Autodesk Fusion 360 part; units mm, degrees
note: some values were not read from the file. Set by a fixed rule: the direction of a hole.
(part 5 of 10)
  line L3822 (47.9298, 29.8196) -> (47.5996, 30.1498)
  line L3823 (47.9298, 31.1404) -> (48.5902, 31.1404)
  line L3824 (48.5902, 29.8196) -> (47.9298, 29.8196)
  line L3825 (48.9204, 30.8102) -> (48.9204, 30.1498)
  line L3826 (48.9204, 30.1498) -> (48.5902, 29.8196)
  line L3827 (48.5902, 31.1404) -> (48.9204, 30.8102)
  line L3828 (52.6796, 20.6502) -> (53.0098, 20.9804)
  line L3829 (53.6702, 19.6596) -> (53.0098, 19.6596)
  line L3830 (52.6796, 19.9898) -> (52.6796, 20.6502)
  line L3831 (54.0004, 20.6502) -> (54.0004, 19.9898)
  line L3832 (53.0098, 20.9804) -> (53.6702, 20.9804)
  line L3833 (53.0098, 19.6596) -> (52.6796, 19.9898)
  line L3834 (53.6702, 20.9804) -> (54.0004, 20.6502)
  line L3835 (54.0004, 19.9898) -> (53.6702, 19.6596)
  line L3836 (53.0098, 31.1404) -> (53.6702, 31.1404)
  line L3837 (54.0004, 30.1498) -> (53.6702, 29.8196)
  line L3838 (54.0004, 30.8102) -> (54.0004, 30.1498)
  line L3839 (53.6702, 31.1404) -> (54.0004, 30.8102)
  line L3840 (52.6796, 30.8102) -> (53.0098, 31.1404)
  line L3841 (53.0098, 29.8196) -> (52.6796, 30.1498)
  line L3842 (52.6796, 30.1498) -> (52.6796, 30.8102)
  line L3843 (53.6702, 29.8196) -> (53.0098, 29.8196)
  line L3844 (66.6496, 19.9898) -> (66.6496, 20.6502)
  line L3845 (67.6402, 20.9804) -> (67.9704, 20.6502)
  line L3846 (67.9704, 20.6502) -> (67.9704, 19.9898)
  line L3847 (67.9704, 19.9898) -> (67.6402, 19.6596)
  line L3848 (66.6496, 20.6502) -> (66.9798, 20.9804)
  line L3849 (66.9798, 19.6596) -> (66.6496, 19.9898)
  line L3850 (67.6402, 19.6596) -> (66.9798, 19.6596)
  line L3851 (66.9798, 20.9804) -> (67.6402, 20.9804)
  line L3852 (66.9798, 31.1404) -> (67.6402, 31.1404)
  line L3853 (67.9704, 30.8102) -> (67.9704, 30.1498)
  line L3854 (67.6402, 31.1404) -> (67.9704, 30.8102)
  line L3855 (66.9798, 29.8196) -> (66.6496, 30.1498)
  line L3856 (67.9704, 30.1498) -> (67.6402, 29.8196)
  line L3857 (66.6496, 30.1498) -> (66.6496, 30.8102)
  line L3858 (66.6496, 30.8102) -> (66.9798, 31.1404)
  line L3859 (67.6402, 29.8196) -> (66.9798, 29.8196)
  line L3860 (78.4098, 20.9804) -> (79.0702, 20.9804)
  line L3861 (79.4004, 19.9898) -> (79.0702, 19.6596)
  line L3862 (79.0702, 19.6596) -> (78.4098, 19.6596)
  line L3863 (79.0702, 20.9804) -> (79.4004, 20.6502)
  line L3864 (79.4004, 20.6502) -> (79.4004, 19.9898)
  line L3865 (78.4098, 19.6596) -> (78.0796, 19.9898)
  line L3866 (78.0796, 19.9898) -> (78.0796, 20.6502)
  line L3867 (78.0796, 20.6502) -> (78.4098, 20.9804)
  line L3868 (79.0702, 29.8196) -> (78.4098, 29.8196)
  line L3869 (79.0702, 31.1404) -> (79.4004, 30.8102)
  line L3870 (79.4004, 30.8102) -> (79.4004, 30.1498)
  line L3871 (78.4098, 29.8196) -> (78.0796, 30.1498)
  line L3872 (78.0796, 30.8102) -> (78.4098, 31.1404)
  line L3873 (78.4098, 31.1404) -> (79.0702, 31.1404)
  line L3874 (79.4004, 30.1498) -> (79.0702, 29.8196)
  line L3875 (78.0796, 30.1498) -> (78.0796, 30.8102)
  line L3876 (90.5002, 19.6596) -> (89.8398, 19.6596)
  line L3877 (90.8304, 19.9898) -> (90.5002, 19.6596)
  line L3878 (89.5096, 19.9898) -> (89.5096, 20.6502)
  line L3879 (89.8398, 20.9804) -> (90.5002, 20.9804)
  line L3880 (90.5002, 20.9804) -> (90.8304, 20.6502)
  line L3881 (89.8398, 19.6596) -> (89.5096, 19.9898)
  line L3882 (90.8304, 20.6502) -> (90.8304, 19.9898)
  line L3883 (89.5096, 20.6502) -> (89.8398, 20.9804)
  line L3884 (89.5096, 30.1498) -> (89.5096, 30.8102)
  line L3885 (89.5096, 30.8102) -> (89.8398, 31.1404)
  line L3886 (89.8398, 31.1404) -> (90.5002, 31.1404)
  line L3887 (90.8304, 30.8102) -> (90.8304, 30.1498)
  line L3888 (90.8304, 30.1498) -> (90.5002, 29.8196)
  line L3889 (90.5002, 29.8196) -> (89.8398, 29.8196)
  line L3890 (89.8398, 29.8196) -> (89.5096, 30.1498)
  line L3891 (90.5002, 31.1404) -> (90.8304, 30.8102)
  line L3892 (34.7234, 76.3657) -> (34.2565, 76.8326)
  line L3893 (35.6574, 76.8326) -> (35.1904, 76.3657)
  line L3894 (34.2565, 76.8326) -> (34.2565, 77.2996)
  line L3895 (35.1904, 77.7666) -> (35.6574, 77.2996)
  line L3896 (35.1904, 76.3657) -> (34.7234, 76.3657)
  line L3897 (34.2565, 77.2996) -> (34.7234, 77.7666)
  line L3898 (34.7234, 77.7666) -> (35.1904, 77.7666)
  line L3899 (35.6574, 77.2996) -> (35.6574, 76.8326)
  line L3900 (41.9076, 69.1815) -> (41.4407, 69.6484)
  line L3901 (41.4407, 69.6484) -> (41.4407, 70.1154)
  line L3902 (42.3746, 70.5824) -> (42.8416, 70.1154)
  line L3903 (42.8416, 70.1154) -> (42.8416, 69.6484)
  line L3904 (42.3746, 69.1815) -> (41.9076, 69.1815)
  line L3905 (41.4407, 70.1154) -> (41.9076, 70.5824)
  line L3906 (42.8416, 69.6484) -> (42.3746, 69.1815)
  line L3907 (41.9076, 70.5824) -> (42.3746, 70.5824)
  line L3908 (28.5496, 77.1652) -> (28.8798, 77.4954)
  line L3909 (28.8798, 76.1746) -> (28.5496, 76.5048)
  line L3910 (28.8798, 77.4954) -> (29.5402, 77.4954)
  line L3911 (28.5496, 76.5048) -> (28.5496, 77.1652)
  line L3912 (29.8704, 77.1652) -> (29.8704, 76.5048)
  line L3913 (29.5402, 76.1746) -> (28.8798, 76.1746)
  line L3914 (29.5402, 77.4954) -> (29.8704, 77.1652)
  line L3915 (29.8704, 76.5048) -> (29.5402, 76.1746)
  line L3916 (27.0002, 76.1746) -> (26.3398, 76.1746)
  line L3917 (26.3398, 76.1746) -> (26.0096, 76.5048)
  line L3918 (27.3304, 76.5048) -> (27.0002, 76.1746)
  line L3919 (26.0096, 77.1652) -> (26.3398, 77.4954)
  line L3920 (26.3398, 77.4954) -> (27.0002, 77.4954)
  line L3921 (27.0002, 77.4954) -> (27.3304, 77.1652)
  line L3922 (27.3304, 77.1652) -> (27.3304, 76.5048)
  line L3923 (26.0096, 76.5048) -> (26.0096, 77.1652)
  line L3924 (88.265, 70.485) -> (75.565, 57.785)
  line L3925 (98.425, 37.465) -> (98.425, 70.485)
  line L3926 (52.07, 57.785) -> (52.07, 37.465)
  line L3927 (75.565, 57.785) -> (52.07, 57.785)
  line L3928 (52.07, 37.465) -> (98.425, 37.465)
  line L3929 (98.425, 70.485) -> (88.265, 70.485)
  line L3930 (1.27, 71.12) -> (10.795, 71.12)
  line L3931 (1.27, 37.465) -> (1.27, 71.12)
  line L3932 (10.795, 71.12) -> (24.13, 57.785)
  line L3933 (48.895, 57.785) -> (48.895, 37.465)
  line L3934 (48.895, 37.465) -> (1.27, 37.465)
  line L3935 (24.13, 57.785) -> (48.895, 57.785)
  line L3936 (74.295, 70.485) -> (66.04, 78.74)
  line L3937 (26.035, 59.69) -> (74.295, 59.69)
  line L3938 (74.295, 59.69) -> (74.295, 70.485)
  line L3939 (66.04, 78.74) -> (34.29, 78.74)
  line L3940 (34.29, 78.74) -> (26.035, 70.485)
  line L3941 (26.035, 70.485) -> (26.035, 59.69)
  line L3942 (52.1716, 57.6834) -> (75.565, 57.6834)
  line L3943 (75.565, 57.6834) -> (75.6039, 57.6911)
  line L3944 (95.575, 66.9873) -> (95.3582, 66.5617)
  line L3945 (97.8163, 62.4021) -> (98.1561, 62.83)
  line L3946 (96.81, 67.6165) -> (96.3383, 67.5418)
  line L3947 (75.6039, 57.6911) -> (75.6368, 57.7132)
  line L3948 (96.3383, 67.5418) -> (95.9127, 67.325)
  line L3949 (95.2835, 66.09) -> (95.2835, 66.09)
  line L3950 (52.1716, 37.5666) -> (52.1716, 57.6834)
  line L3951 (95.2835, 63.55) -> (95.2835, 63.55)
  line L3952 (88.3071, 70.3834) -> (98.3234, 70.3834)
  line L3953 (98.1561, 66.81) -> (97.8163, 67.2379)
  line L3954 (98.3234, 63.3501) -> (98.3234, 37.5666)
  line L3955 (98.1561, 62.83) -> (98.3234, 63.3501)
  line L3956 (95.2835, 66.09) -> (95.2835, 63.55)
  line L3957 (75.6368, 57.7132) -> (88.3071, 70.3834)
  line L3958 (95.3582, 66.5617) -> (95.2835, 66.09)
  line L3959 (95.9127, 62.315) -> (96.3383, 62.0982)
  line L3960 (95.3582, 63.0783) -> (95.575, 62.6527)
  line L3961 (96.3383, 62.0982) -> (96.81, 62.0235)
  line L3962 (95.2835, 63.55) -> (95.3582, 63.0783)
  line L3963 (98.3234, 37.5666) -> (52.1716, 37.5666)
  line L3964 (97.8163, 67.2379) -> (97.3476, 67.5188)
  line L3965 (97.3476, 62.1212) -> (97.8163, 62.4021)
  line L3966 (98.3234, 70.3834) -> (98.3234, 66.2899)
  line L3967 (98.3234, 66.2899) -> (98.1561, 66.81)
  line L3968 (75.6368, 57.7132) -> (75.6368, 57.7132)
  line L3969 (97.3476, 67.5188) -> (96.81, 67.6165)
  line L3970 (95.575, 62.6527) -> (95.9127, 62.315)
  line L3971 (95.9127, 67.325) -> (95.575, 66.9873)
  line L3972 (96.81, 62.0235) -> (97.3476, 62.1212)
  line L3973 (95.813, 56.2555) -> (95.813, 56.2555)
  line L3974 (93.273, 56.2555) -> (93.273, 56.2555)
  line L3975 (92.038, 55.6263) -> (91.8212, 55.2007)
  line L3976 (95.813, 53.2025) -> (96.2847, 53.2772)
  line L3977 (92.3757, 55.964) -> (92.038, 55.6263)
  line L3978 (91.8212, 54.2573) -> (92.038, 53.8317)
  line L3979 (93.273, 53.2025) -> (93.273, 53.2025)
  line L3980 (95.813, 53.2025) -> (95.813, 53.2025)
  line L3981 (96.7103, 55.964) -> (96.2847, 56.1808)
  line L3982 (91.7465, 54.729) -> (91.8212, 54.2573)
  line L3983 (95.813, 56.2555) -> (93.273, 56.2555)
  line L3984 (91.8212, 55.2007) -> (91.7465, 54.729)
  line L3985 (96.7103, 53.494) -> (97.048, 53.8317)
  line L3986 (92.8013, 56.1808) -> (92.3757, 55.964)
  line L3987 (97.2648, 55.2007) -> (97.048, 55.6263)
  line L3988 (97.2648, 54.2573) -> (97.3395, 54.729)
  line L3989 (93.273, 53.2025) -> (95.813, 53.2025)
  line L3990 (92.8013, 53.2772) -> (93.273, 53.2025)
  line L3991 (96.2847, 56.1808) -> (95.813, 56.2555)
  line L3992 (92.3757, 53.494) -> (92.8013, 53.2772)
  line L3993 (97.3395, 54.729) -> (97.2648, 55.2007)
  line L3994 (96.2847, 53.2772) -> (96.7103, 53.494)
  line L3995 (97.048, 55.6263) -> (96.7103, 55.964)
  line L3996 (93.273, 56.2555) -> (92.8013, 56.1808)
  line L3997 (97.048, 53.8317) -> (97.2648, 54.2573)
  line L3998 (92.038, 53.8317) -> (92.3757, 53.494)
  line L3999 (71.5197, 53.2772) -> (71.9453, 53.494)
  line L4000 (71.048, 53.2025) -> (71.5197, 53.2772)
  line L4001 (71.048, 53.2025) -> (71.048, 53.2025)
  line L4002 (71.5197, 56.1808) -> (71.048, 56.2555)
  line L4003 (68.0363, 53.2772) -> (68.508, 53.2025)
  line L4004 (67.0562, 54.2573) -> (67.273, 53.8317)
  line L4005 (67.6107, 55.964) -> (67.273, 55.6263)
  line L4006 (68.508, 56.2555) -> (68.0363, 56.1808)
  line L4007 (72.283, 53.8317) -> (72.4998, 54.2573)
  line L4008 (72.4998, 55.2007) -> (72.283, 55.6263)
  line L4009 (72.4998, 54.2573) -> (72.5745, 54.729)
  line L4010 (71.048, 56.2555) -> (68.508, 56.2555)
  line L4011 (72.5745, 54.729) -> (72.4998, 55.2007)
  line L4012 (71.9453, 53.494) -> (72.283, 53.8317)
  line L4013 (67.273, 53.8317) -> (67.6107, 53.494)
  line L4014 (66.9815, 54.729) -> (67.0562, 54.2573)
  line L4015 (68.508, 53.2025) -> (68.508, 53.2025)
  line L4016 (72.283, 55.6263) -> (71.9453, 55.964)
  line L4017 (71.048, 56.2555) -> (71.048, 56.2555)
  line L4018 (67.273, 55.6263) -> (67.0562, 55.2007)
  line L4019 (67.0562, 55.2007) -> (66.9815, 54.729)
  line L4020 (68.0363, 56.1808) -> (67.6107, 55.964)
  line L4021 (67.6107, 53.494) -> (68.0363, 53.2772)
  line L4022 (68.508, 56.2555) -> (68.508, 56.2555)
  line L4023 (68.508, 53.2025) -> (71.048, 53.2025)
  line L4024 (71.9453, 55.964) -> (71.5197, 56.1808)
  line L4025 (79.7562, 54.2573) -> (79.973, 53.8317)
  line L4026 (84.6453, 55.964) -> (84.2197, 56.1808)
  line L4027 (85.1998, 54.2573) -> (85.2745, 54.729)
  line L4028 (83.748, 53.2025) -> (84.2197, 53.2772)
  line L4029 (84.983, 53.8317) -> (85.1998, 54.2573)
  line L4030 (81.208, 56.2555) -> (80.7363, 56.1808)
  line L4031 (80.7363, 53.2772) -> (81.208, 53.2025)
  line L4032 (80.3107, 53.494) -> (80.7363, 53.2772)
  line L4033 (84.983, 55.6263) -> (84.6453, 55.964)
  line L4034 (81.208, 56.2555) -> (81.208, 56.2555)
  line L4035 (81.208, 53.2025) -> (81.208, 53.2025)
  line L4036 (79.973, 53.8317) -> (80.3107, 53.494)
  line L4037 (79.7562, 55.2007) -> (79.6815, 54.729)
  line L4038 (81.208, 53.2025) -> (83.748, 53.2025)
  line L4039 (83.748, 53.2025) -> (83.748, 53.2025)
  line L4040 (79.6815, 54.729) -> (79.7562, 54.2573)
  line L4041 (84.2197, 56.1808) -> (83.748, 56.2555)
  line L4042 (85.1998, 55.2007) -> (84.983, 55.6263)
  line L4043 (83.748, 56.2555) -> (81.208, 56.2555)
  line L4044 (80.7363, 56.1808) -> (80.3107, 55.964)
  line L4045 (84.6453, 53.494) -> (84.983, 53.8317)
  line L4046 (80.3107, 55.964) -> (79.973, 55.6263)
  line L4047 (83.748, 56.2555) -> (83.748, 56.2555)
  line L4048 (79.973, 55.6263) -> (79.7562, 55.2007)
  line L4049 (84.2197, 53.2772) -> (84.6453, 53.494)
  line L4050 (85.2745, 54.729) -> (85.1998, 55.2007)
  line L4051 (58.348, 56.2555) -> (58.348, 56.2555)
  line L4052 (59.583, 55.6263) -> (59.2453, 55.964)
  line L4053 (55.3363, 53.2772) -> (55.808, 53.2025)
  line L4054 (54.3562, 54.2573) -> (54.573, 53.8317)
  line L4055 (55.808, 56.2555) -> (55.3363, 56.1808)
  line L4056 (58.348, 53.2025) -> (58.348, 53.2025)
  line L4057 (59.7998, 55.2007) -> (59.583, 55.6263)
  line L4058 (59.8745, 54.729) -> (59.7998, 55.2007)
  line L4059 (59.583, 53.8317) -> (59.7998, 54.2573)
  line L4060 (59.2453, 53.494) -> (59.583, 53.8317)
  line L4061 (58.8197, 53.2772) -> (59.2453, 53.494)
  line L4062 (58.348, 53.2025) -> (58.8197, 53.2772)
  line L4063 (55.808, 53.2025) -> (55.808, 53.2025)
  line L4064 (59.7998, 54.2573) -> (59.8745, 54.729)
  line L4065 (54.573, 55.6263) -> (54.3562, 55.2007)
  line L4066 (59.2453, 55.964) -> (58.8197, 56.1808)
  line L4067 (58.348, 56.2555) -> (55.808, 56.2555)
  line L4068 (55.808, 56.2555) -> (55.808, 56.2555)
  line L4069 (54.573, 53.8317) -> (54.9107, 53.494)
  line L4070 (55.808, 53.2025) -> (58.348, 53.2025)
  line L4071 (58.8197, 56.1808) -> (58.348, 56.2555)
  line L4072 (54.3562, 55.2007) -> (54.2815, 54.729)
  line L4073 (54.9107, 53.494) -> (55.3363, 53.2772)
  line L4074 (54.2815, 54.729) -> (54.3562, 54.2573)
  line L4075 (54.9107, 55.964) -> (54.573, 55.6263)
  line L4076 (55.3363, 56.1808) -> (54.9107, 55.964)
  line L4077 (1.3716, 71.0184) -> (10.7529, 71.0184)
  line L4078 (48.7934, 57.6834) -> (48.7934, 37.5666)
  line L4079 (24.0582, 57.7132) -> (24.0582, 57.7132)
  line L4080 (24.13, 57.6834) -> (48.7934, 57.6834)
  line L4081 (24.0911, 57.6911) -> (24.13, 57.6834)
  line L4082 (1.3716, 37.5666) -> (1.3716, 71.0184)
  line L4083 (24.0582, 57.7132) -> (24.0911, 57.6911)
  line L4084 (48.7934, 37.5666) -> (1.3716, 37.5666)
  line L4085 (10.7529, 71.0184) -> (24.0582, 57.7132)
  line L4086 (2.9212, 54.2573) -> (3.138, 53.8317)
  line L4087 (3.9013, 53.2772) -> (4.373, 53.2025)
  line L4088 (6.913, 53.2025) -> (7.3847, 53.2772)
  line L4089 (3.138, 53.8317) -> (3.4757, 53.494)
  line L4090 (2.8465, 54.729) -> (2.9212, 54.2573)
  line L4091 (4.373, 53.2025) -> (4.373, 53.2025)
  line L4092 (3.9013, 56.1808) -> (3.4757, 55.964)
  line L4093 (3.138, 55.6263) -> (2.9212, 55.2007)
  line L4094 (7.3847, 56.1808) -> (6.913, 56.2555)
  line L4095 (3.4757, 53.494) -> (3.9013, 53.2772)
  line L4096 (2.9212, 55.2007) -> (2.8465, 54.729)
  line L4097 (6.913, 53.2025) -> (6.913, 53.2025)
  line L4098 (7.8103, 53.494) -> (8.148, 53.8317)
  line L4099 (6.913, 56.2555) -> (4.373, 56.2555)
  line L4100 (8.3648, 55.2007) -> (8.148, 55.6263)
  line L4101 (8.148, 55.6263) -> (7.8103, 55.964)
  line L4102 (7.8103, 55.964) -> (7.3847, 56.1808)
  line L4103 (8.148, 53.8317) -> (8.3648, 54.2573)
  line L4104 (6.913, 56.2555) -> (6.913, 56.2555)
  line L4105 (3.4757, 55.964) -> (3.138, 55.6263)
  line L4106 (8.3648, 54.2573) -> (8.4395, 54.729)
  line L4107 (4.373, 56.2555) -> (3.9013, 56.1808)
  line L4108 (4.373, 56.2555) -> (4.373, 56.2555)
  line L4109 (7.3847, 53.2772) -> (7.8103, 53.494)
  line L4110 (4.373, 53.2025) -> (6.913, 53.2025)
  line L4111 (8.4395, 54.729) -> (8.3648, 55.2007)
  line L4112 (20.848, 55.6263) -> (20.5103, 55.964)
  line L4113 (21.1395, 54.729) -> (21.0648, 55.2007)
  line L4114 (20.5103, 55.964) -> (20.0847, 56.1808)
  line L4115 (20.0847, 56.1808) -> (19.613, 56.2555)
  line L4116 (19.613, 56.2555) -> (19.613, 56.2555)
  line L4117 (20.848, 53.8317) -> (21.0648, 54.2573)
  line L4118 (21.0648, 54.2573) -> (21.1395, 54.729)
  line L4119 (15.6212, 54.2573) -> (15.838, 53.8317)
  line L4120 (19.613, 56.2555) -> (17.073, 56.2555)
  line L4121 (17.073, 56.2555) -> (17.073, 56.2555)
  line L4122 (15.5465, 54.729) -> (15.6212, 54.2573)
  line L4123 (15.838, 55.6263) -> (15.6212, 55.2007)
  line L4124 (21.0648, 55.2007) -> (20.848, 55.6263)
  line L4125 (16.1757, 55.964) -> (15.838, 55.6263)
  line L4126 (16.6013, 53.2772) -> (17.073, 53.2025)
  line L4127 (17.073, 56.2555) -> (16.6013, 56.1808)
  line L4128 (16.1757, 53.494) -> (16.6013, 53.2772)
  line L4129 (15.6212, 55.2007) -> (15.5465, 54.729)
  line L4130 (17.073, 53.2025) -> (17.073, 53.2025)
  line L4131 (19.613, 53.2025) -> (20.0847, 53.2772)
  line L4132 (19.613, 53.2025) -> (19.613, 53.2025)
  line L4133 (15.838, 53.8317) -> (16.1757, 53.494)
  line L4134 (16.6013, 56.1808) -> (16.1757, 55.964)
  line L4135 (17.073, 53.2025) -> (19.613, 53.2025)
  line L4136 (20.5103, 53.494) -> (20.848, 53.8317)
  line L4137 (20.0847, 53.2772) -> (20.5103, 53.494)
  line L4138 (32.7847, 53.2772) -> (33.2103, 53.494)
  line L4139 (33.2103, 53.494) -> (33.548, 53.8317)
  line L4140 (33.548, 55.6263) -> (33.2103, 55.964)
  line L4141 (29.773, 53.2025) -> (29.773, 53.2025)
  line L4142 (32.313, 53.2025) -> (32.313, 53.2025)
  line L4143 (29.773, 56.2555) -> (29.3013, 56.1808)
  line L4144 (32.7847, 56.1808) -> (32.313, 56.2555)
  line L4145 (28.538, 53.8317) -> (28.8757, 53.494)
  line L4146 (32.313, 56.2555) -> (29.773, 56.2555)
  line L4147 (28.8757, 55.964) -> (28.538, 55.6263)
  line L4148 (28.8757, 53.494) -> (29.3013, 53.2772)
  line L4149 (33.548, 53.8317) -> (33.7648, 54.2573)
  line L4150 (28.3212, 55.2007) -> (28.2465, 54.729)
  line L4151 (32.313, 56.2555) -> (32.313, 56.2555)
  line L4152 (33.7648, 55.2007) -> (33.548, 55.6263)
  line L4153 (33.2103, 55.964) -> (32.7847, 56.1808)
  line L4154 (29.3013, 56.1808) -> (28.8757, 55.964)
  line L4155 (28.3212, 54.2573) -> (28.538, 53.8317)
  line L4156 (32.313, 53.2025) -> (32.7847, 53.2772)
  line L4157 (29.773, 56.2555) -> (29.773, 56.2555)
  line L4158 (33.7648, 54.2573) -> (33.8395, 54.729)
  line L4159 (33.8395, 54.729) -> (33.7648, 55.2007)
  line L4160 (28.538, 55.6263) -> (28.3212, 55.2007)
  line L4161 (28.2465, 54.729) -> (28.3212, 54.2573)
  line L4162 (29.3013, 53.2772) -> (29.773, 53.2025)
  line L4163 (29.773, 53.2025) -> (32.313, 53.2025)
  line L4164 (4.9718, 62.9783) -> (5.0465, 63.45)
  line L4165 (4.755, 62.5527) -> (4.9718, 62.9783)
  line L4166 (4.4173, 62.215) -> (4.755, 62.5527)
  line L4167 (3.9917, 61.9982) -> (4.4173, 62.215)
  line L4168 (3.0483, 61.9982) -> (3.52, 61.9235)
  line L4169 (3.52, 67.5165) -> (3.0483, 67.4418)
  line L4170 (5.0465, 63.45) -> (5.0465, 63.45)
  line L4171 (3.9917, 67.4418) -> (3.52, 67.5165)
  line L4172 (5.0465, 63.45) -> (5.0465, 65.99)
  line L4173 (3.52, 61.9235) -> (3.9917, 61.9982)
  line L4174 (1.9935, 63.45) -> (2.0682, 62.9783)
  line L4175 (5.0465, 65.99) -> (5.0465, 65.99)
  line L4176 (2.6227, 62.215) -> (3.0483, 61.9982)
  line L4177 (3.0483, 67.4418) -> (2.6227, 67.225)
  line L4178 (2.285, 62.5527) -> (2.6227, 62.215)
  line L4179 (4.4173, 67.225) -> (3.9917, 67.4418)
  line L4180 (1.9935, 63.45) -> (1.9935, 63.45)
  line L4181 (5.0465, 65.99) -> (4.9718, 66.4617)
  line L4182 (2.0682, 62.9783) -> (2.285, 62.5527)
  line L4183 (4.9718, 66.4617) -> (4.755, 66.8873)
  line L4184 (2.0682, 66.4617) -> (1.9935, 65.99)
  line L4185 (4.755, 66.8873) -> (4.4173, 67.225)
  line L4186 (2.285, 66.8873) -> (2.0682, 66.4617)
  line L4187 (1.9935, 65.99) -> (1.9935, 63.45)
  line L4188 (2.6227, 67.225) -> (2.285, 66.8873)
  line L4189 (1.9935, 65.99) -> (1.9935, 65.99)
  line L4190 (45.013, 56.2555) -> (45.013, 56.2555)
  line L4191 (45.013, 53.2025) -> (45.013, 53.2025)
  line L4192 (41.0212, 55.2007) -> (40.9465, 54.729)
  line L4193 (41.238, 53.8317) -> (41.5757, 53.494)
  line L4194 (46.5395, 54.729) -> (46.4648, 55.2007)
  line L4195 (42.473, 56.2555) -> (42.473, 56.2555)
  line L4196 (41.0212, 54.2573) -> (41.238, 53.8317)
  line L4197 (40.9465, 54.729) -> (41.0212, 54.2573)
  line L4198 (42.0013, 56.1808) -> (41.5757, 55.964)
  line L4199 (46.4648, 54.2573) -> (46.5395, 54.729)
  line L4200 (46.4648, 55.2007) -> (46.248, 55.6263)
  line L4201 (41.5757, 53.494) -> (42.0013, 53.2772)
  line L4202 (41.238, 55.6263) -> (41.0212, 55.2007)
  line L4203 (41.5757, 55.964) -> (41.238, 55.6263)
  line L4204 (46.248, 55.6263) -> (45.9103, 55.964)
  line L4205 (42.473, 53.2025) -> (45.013, 53.2025)
  line L4206 (45.4847, 53.2772) -> (45.9103, 53.494)
  line L4207 (42.473, 53.2025) -> (42.473, 53.2025)
  line L4208 (46.248, 53.8317) -> (46.4648, 54.2573)
  line L4209 (45.9103, 53.494) -> (46.248, 53.8317)
  line L4210 (42.0013, 53.2772) -> (42.473, 53.2025)
  line L4211 (42.473, 56.2555) -> (42.0013, 56.1808)
  line L4212 (45.013, 53.2025) -> (45.4847, 53.2772)
  line L4213 (45.9103, 55.964) -> (45.4847, 56.1808)
  line L4214 (45.013, 56.2555) -> (42.473, 56.2555)
  line L4215 (45.4847, 56.1808) -> (45.013, 56.2555)
  line L4216 (34.5864, 78.0975) -> (34.4702, 78.0198)
  line L4217 (34.0032, 77.5528) -> (34.0032, 77.5528)
  line L4218 (34.5864, 76.0348) -> (34.7234, 76.0075)
  line L4219 (26.1366, 59.7916) -> (26.1366, 70.4429)
  line L4220 (35.3275, 78.0975) -> (35.1904, 78.1247)
  line L4221 (34.4702, 78.0198) -> (34.4702, 78.0198)
  line L4222 (65.9979, 78.6384) -> (74.1934, 70.4429)
  line L4223 (35.9882, 76.6956) -> (36.0155, 76.8326)
  line L4224 (34.1819, 76.4007) -> (34.4702, 76.1124)
  line L4225 (36.0155, 77.2996) -> (35.9882, 77.4367)
  line L4226 (35.1904, 76.0075) -> (35.3275, 76.0348)
  line L4227 (35.9106, 77.5528) -> (35.4436, 78.0198)
  line L4228 (35.1904, 78.1247) -> (34.7234, 78.1247)
  line L4229 (26.1366, 70.4429) -> (32.0943, 76.4007)
  line L4230 (35.9106, 77.5528) -> (35.9106, 77.5528)
  line L4231 (35.4436, 78.0198) -> (35.3275, 78.0975)
  line L4232 (35.1904, 76.0075) -> (35.1904, 76.0075)
  line L4233 (34.4702, 76.1124) -> (34.4702, 76.1124)
  line L4234 (33.8983, 77.2996) -> (33.8983, 77.2996)
  line L4235 (34.7234, 76.0075) -> (34.7234, 76.0075)
  line L4236 (34.7234, 76.0075) -> (35.1904, 76.0075)
  line L4237 (36.0155, 77.2996) -> (36.0155, 77.2996)
  line L4238 (35.3275, 76.0348) -> (35.4436, 76.1124)
  line L4239 (74.1934, 59.7916) -> (26.1366, 59.7916)
  line L4240 (32.0943, 76.4007) -> (34.1819, 76.4007)
  line L4241 (74.1934, 70.4429) -> (74.1934, 59.7916)
  line L4242 (36.0155, 76.8326) -> (36.0155, 76.8326)
  line L4243 (34.4702, 76.1124) -> (34.5864, 76.0348)
  line L4244 (35.9106, 76.5794) -> (35.9106, 76.5794)
  line L4245 (35.4436, 78.0198) -> (35.4436, 78.0198)
  line L4246 (35.9882, 77.4367) -> (35.9106, 77.5528)
  line L4247 (33.9256, 77.4367) -> (33.8983, 77.2996)
  line L4248 (35.4436, 76.1124) -> (35.9106, 76.5794)
  line L4249 (34.4702, 78.0198) -> (34.0032, 77.5528)
  line L4250 (35.9106, 76.5794) -> (35.9882, 76.6956)
  line L4251 (33.8983, 77.2693) -> (32.963, 77.2693)
  line L4252 (36.0155, 76.8326) -> (36.0155, 77.2996)
  line L4253 (33.8983, 77.2996) -> (33.8983, 77.2693)
  line L4254 (32.963, 77.2693) -> (34.3321, 78.6384)
  line L4255 (34.0032, 77.5528) -> (33.9256, 77.4367)
  line L4256 (34.7234, 78.1247) -> (34.7234, 78.1247)
  line L4257 (35.1904, 78.1247) -> (35.1904, 78.1247)
  line L4258 (34.7234, 78.1247) -> (34.5864, 78.0975)
  line L4259 (34.3321, 78.6384) -> (65.9979, 78.6384)
  line L4260 (38.5465, 65.965) -> (38.4718, 66.4367)
  line L4261 (35.5682, 66.4367) -> (35.4935, 65.965)
  line L4262 (37.4917, 61.9732) -> (37.9173, 62.19)
  line L4263 (38.5465, 65.965) -> (38.5465, 65.965)
  line L4264 (36.1227, 67.2) -> (35.785, 66.8623)
  line L4265 (35.4935, 65.965) -> (35.4935, 63.425)
  line L4266 (38.255, 62.5277) -> (38.4718, 62.9533)
  line L4267 (37.02, 67.4915) -> (36.5483, 67.4168)
  line L4268 (36.5483, 61.9732) -> (37.02, 61.8985)
  line L4269 (35.4935, 63.425) -> (35.4935, 63.425)
  line L4270 (35.785, 66.8623) -> (35.5682, 66.4367)
  line L4271 (36.5483, 67.4168) -> (36.1227, 67.2)
  line L4272 (35.785, 62.5277) -> (36.1227, 62.19)
  line L4273 (35.4935, 65.965) -> (35.4935, 65.965)
  line L4274 (38.5465, 63.425) -> (38.5465, 63.425)
  line L4275 (35.4935, 63.425) -> (35.5682, 62.9533)
  line L4276 (38.5465, 63.425) -> (38.5465, 65.965)
  line L4277 (38.255, 66.8623) -> (37.9173, 67.2)
  line L4278 (37.4917, 67.4168) -> (37.02, 67.4915)
  line L4279 (36.1227, 62.19) -> (36.5483, 61.9732)
  line L4280 (38.4718, 62.9533) -> (38.5465, 63.425)
  line L4281 (37.9173, 62.19) -> (38.255, 62.5277)
  line L4282 (37.9173, 67.2) -> (37.4917, 67.4168)
  line L4283 (35.5682, 62.9533) -> (35.785, 62.5277)
  line L4284 (37.02, 61.8985) -> (37.4917, 61.9732)
  line L4285 (38.4718, 66.4367) -> (38.255, 66.8623)
  line L4286 (61.8582, 63.1033) -> (62.075, 62.6777)
  line L4287 (64.7618, 63.1033) -> (64.8365, 63.575)
  line L4288 (61.7835, 63.575) -> (61.8582, 63.1033)
  line L4289 (62.075, 62.6777) -> (62.4127, 62.34)
  line L4290 (63.31, 67.6415) -> (62.8383, 67.5668)
  line L4291 (63.7817, 67.5668) -> (63.31, 67.6415)
  line L4292 (61.7835, 66.115) -> (61.7835, 63.575)
  line L4293 (63.31, 62.0485) -> (63.7817, 62.1232)
  line L4294 (63.7817, 62.1232) -> (64.2073, 62.34)
  line L4295 (64.7618, 66.5867) -> (64.545, 67.0123)
  line L4296 (61.7835, 63.575) -> (61.7835, 63.575)
  line L4297 (64.2073, 67.35) -> (63.7817, 67.5668)
  line L4298 (62.4127, 67.35) -> (62.075, 67.0123)
  line L4299 (62.075, 67.0123) -> (61.8582, 66.5867)
  line L4300 (61.7835, 66.115) -> (61.7835, 66.115)
  line L4301 (64.545, 62.6777) -> (64.7618, 63.1033)
  line L4302 (64.545, 67.0123) -> (64.2073, 67.35)
  line L4303 (61.8582, 66.5867) -> (61.7835, 66.115)
  line L4304 (62.4127, 62.34) -> (62.8383, 62.1232)
  line L4305 (64.8365, 63.575) -> (64.8365, 66.115)
  line L4306 (64.8365, 66.115) -> (64.8365, 66.115)
  line L4307 (62.8383, 62.1232) -> (63.31, 62.0485)
  line L4308 (62.8383, 67.5668) -> (62.4127, 67.35)
  line L4309 (64.8365, 63.575) -> (64.8365, 63.575)
  line L4310 (64.2073, 62.34) -> (64.545, 62.6777)
  line L4311 (64.8365, 66.115) -> (64.7618, 66.5867)
  line L4312 (52.0008, 76.8601) -> (51.9319, 76.425)
  line L4313 (54.1677, 73.1858) -> (54.4792, 73.4973)
  line L4314 (54.4792, 77.2527) -> (54.1677, 77.5642)
  line L4315 (52.5123, 73.1858) -> (52.9049, 72.9858)
  line L4316 (52.9049, 72.9858) -> (53.34, 72.9169)
  line L4317 (54.7481, 76.425) -> (54.7481, 76.425)
  line L4318 (52.5123, 77.5642) -> (52.2008, 77.2527)
  line L4319 (54.7481, 74.325) -> (54.7481, 76.425)
  line L4320 (54.1677, 77.5642) -> (53.7751, 77.7642)
  line L4321 (51.9319, 76.425) -> (51.9319, 76.425)
  line L4322 (54.7481, 76.425) -> (54.6792, 76.8601)
  line L4323 (54.4792, 73.4973) -> (54.6792, 73.8899)
  line L4324 (51.9319, 74.325) -> (51.9319, 74.325)
  line L4325 (53.34, 72.9169) -> (53.7751, 72.9858)
  line L4326 (52.2008, 77.2527) -> (52.0008, 76.8601)
  line L4327 (51.9319, 76.425) -> (51.9319, 74.325)
  line L4328 (53.7751, 77.7642) -> (53.34, 77.8331)
  line L4329 (51.9319, 74.325) -> (52.0008, 73.8899)
  line L4330 (54.6792, 73.8899) -> (54.7481, 74.325)
  line L4331 (53.7751, 72.9858) -> (54.1677, 73.1858)
  line L4332 (52.2008, 73.4973) -> (52.5123, 73.1858)
  line L4333 (53.34, 77.8331) -> (52.9049, 77.7642)
  line L4334 (54.6792, 76.8601) -> (54.4792, 77.2527)
  line L4335 (52.0008, 73.8899) -> (52.2008, 73.4973)
  line L4336 (54.7481, 74.325) -> (54.7481, 74.325)
  line L4337 (52.9049, 77.7642) -> (52.5123, 77.5642)
  line L4338 (49.4671, 76.925) -> (49.1839, 77.3489)
  line L4339 (48.76, 77.6321) -> (48.26, 77.7315)
  line L4340 (47.3361, 77.3489) -> (47.0529, 76.925)
  line L4341 (46.9535, 76.425) -> (46.9535, 74.325)
  line L4342 (48.26, 73.0185) -> (48.76, 73.1179)
  line L4343 (49.5665, 74.325) -> (49.5665, 74.325)
  line L4344 (49.1839, 73.4011) -> (49.4671, 73.825)
  line L4345 (49.4671, 73.825) -> (49.5665, 74.325)
  line L4346 (48.26, 77.7315) -> (47.76, 77.6321)
  line L4347 (47.3361, 73.4011) -> (47.76, 73.1179)
  line L4348 (46.9535, 74.325) -> (46.9535, 74.325)
  line L4349 (46.9535, 76.425) -> (46.9535, 76.425)
  line L4350 (46.9535, 74.325) -> (47.0529, 73.825)
  line L4351 (47.0529, 73.825) -> (47.3361, 73.4011)
  line L4352 (47.76, 77.6321) -> (47.3361, 77.3489)
  line L4353 (47.0529, 76.925) -> (46.9535, 76.425)
  line L4354 (49.1839, 77.3489) -> (48.76, 77.6321)
  line L4355 (49.5665, 76.425) -> (49.5665, 76.425)
  line L4356 (47.76, 73.1179) -> (48.26, 73.0185)
  line L4357 (49.5665, 74.325) -> (49.5665, 76.425)
  line L4358 (48.76, 73.1179) -> (49.1839, 73.4011)
  line L4359 (49.5665, 76.425) -> (49.4671, 76.925)
  line L4360 (41.9076, 70.8389) -> (41.9076, 70.8389)
  line L4361 (41.1841, 70.1154) -> (41.1841, 69.6484)
  line L4362 (41.2593, 70.2968) -> (41.2593, 70.2968)
  line L4363 (43.0981, 69.6484) -> (43.0981, 69.6484)
  line L4364 (43.023, 70.2968) -> (43.023, 70.2968)
  line L4365 (42.556, 69) -> (43.023, 69.467)
  line L4366 (41.7262, 69) -> (41.8095, 68.9444)
  line L4367 (41.8095, 68.9444) -> (41.9076, 68.9249)
  line L4368 (41.8095, 70.8194) -> (41.7262, 70.7638)
  line L4369 (41.7262, 70.7638) -> (41.2593, 70.2968)
  line L4370 (43.0786, 69.5502) -> (43.0981, 69.6484)
  line L4371 (42.4728, 70.8194) -> (42.3746, 70.8389)
  line L4372 (43.0981, 70.1154) -> (43.0981, 70.1154)
  line L4373 (42.556, 70.7638) -> (42.556, 70.7638)
  line L4374 (41.9076, 68.9249) -> (41.9076, 68.9249)
  line L4375 (41.2593, 69.467) -> (41.7262, 69)
  line L4376 (41.2036, 70.2136) -> (41.1841, 70.1154)
  line L4377 (41.7262, 69) -> (41.7262, 69)
  line L4378 (42.3746, 68.9249) -> (42.4728, 68.9444)
  line L4379 (43.023, 69.467) -> (43.023, 69.467)
  line L4380 (43.0981, 70.1154) -> (43.0786, 70.2136)
  line L4381 (42.556, 69) -> (42.556, 69)
  line L4382 (41.2036, 69.5502) -> (41.2593, 69.467)
  line L4383 (43.023, 70.2968) -> (42.556, 70.7638)
  line L4384 (41.1841, 70.1154) -> (41.1841, 70.1154)
  line L4385 (43.0786, 70.2136) -> (43.023, 70.2968)
  line L4386 (41.1841, 69.6484) -> (41.1841, 69.6484)
  line L4387 (42.4728, 68.9444) -> (42.556, 69)
  line L4388 (41.9076, 70.8389) -> (41.8095, 70.8194)
  line L4389 (42.3746, 70.8389) -> (42.3746, 70.8389)
  line L4390 (41.9076, 68.9249) -> (42.3746, 68.9249)
  line L4391 (41.1841, 69.6484) -> (41.2036, 69.5502)
  line L4392 (42.3746, 70.8389) -> (41.9076, 70.8389)
  line L4393 (43.0981, 69.6484) -> (43.0981, 70.1154)
  line L4394 (41.7262, 70.7638) -> (41.7262, 70.7638)
  line L4395 (42.3746, 68.9249) -> (42.3746, 68.9249)
  line L4396 (42.556, 70.7638) -> (42.4728, 70.8194)
  line L4397 (41.2593, 69.467) -> (41.2593, 69.467)
  line L4398 (41.2593, 70.2968) -> (41.2036, 70.2136)
  line L4399 (43.023, 69.467) -> (43.0786, 69.5502)
  line L4400 (57.078, 54.729) -> (59.7755, 54.729)
  line L4401 (57.078, 54.729) -> (54.3805, 54.729)
  line L4402 (57.078, 54.729) -> (57.078, 53.3015)
  line L4403 (57.078, 54.729) -> (57.078, 56.1565)
  line L4404 (69.778, 54.729) -> (72.4755, 54.729)
  line L4405 (69.778, 54.729) -> (67.0805, 54.729)
  line L4406 (69.778, 54.729) -> (69.778, 53.3015)
  line L4407 (69.778, 54.729) -> (69.778, 56.1565)
  line L4408 (82.478, 54.729) -> (85.1755, 54.729)
  line L4409 (82.478, 54.729) -> (79.7805, 54.729)
  line L4410 (82.478, 54.729) -> (82.478, 53.3015)
  line L4411 (82.478, 54.729) -> (82.478, 56.1565)
  line L4412 (94.543, 54.729) -> (97.2405, 54.729)
  line L4413 (94.543, 54.729) -> (91.8455, 54.729)
  line L4414 (94.543, 54.729) -> (94.543, 53.3015)
  line L4415 (94.543, 54.729) -> (94.543, 56.1565)
  line L4416 (96.81, 64.82) -> (96.81, 67.5175)
  line L4417 (96.81, 64.82) -> (96.81, 62.1225)
  line L4418 (96.81, 64.82) -> (95.3825, 64.82)
  line L4419 (3.52, 64.72) -> (3.52, 62.0225)
  line L4420 (3.52, 64.72) -> (3.52, 67.4175)
  line L4421 (3.52, 64.72) -> (2.0925, 64.72)
  line L4422 (3.52, 64.72) -> (4.9475, 64.72)
  line L4423 (5.643, 54.729) -> (8.3405, 54.729)
  line L4424 (5.643, 54.729) -> (2.9455, 54.729)
  line L4425 (5.643, 54.729) -> (5.643, 53.3015)
  line L4426 (5.643, 54.729) -> (5.643, 56.1565)
  line L4427 (18.343, 54.729) -> (21.0405, 54.729)
  line L4428 (18.343, 54.729) -> (15.6455, 54.729)
  line L4429 (18.343, 54.729) -> (18.343, 53.3015)
  line L4430 (18.343, 54.729) -> (18.343, 56.1565)
  line L4431 (31.043, 54.729) -> (33.7405, 54.729)
  line L4432 (31.043, 54.729) -> (28.3455, 54.729)
  line L4433 (31.043, 54.729) -> (31.043, 53.3015)
  line L4434 (31.043, 54.729) -> (31.043, 56.1565)
  line L4435 (43.743, 54.729) -> (46.4405, 54.729)
  line L4436 (43.743, 54.729) -> (41.0455, 54.729)
  line L4437 (43.743, 54.729) -> (43.743, 53.3015)
  line L4438 (43.743, 54.729) -> (43.743, 56.1565)
  line L4439 (37.02, 64.695) -> (37.02, 61.9975)
  line L4440 (37.02, 64.695) -> (37.02, 67.3925)
  line L4441 (37.02, 64.695) -> (35.5925, 64.695)
  line L4442 (37.02, 64.695) -> (38.4475, 64.695)
  line L4443 (42.1411, 69.8819) -> (41.5628, 70.4602)
  line L4444 (42.1411, 69.8819) -> (42.7194, 69.3036)
  line L4445 (42.1411, 69.8819) -> (42.7194, 70.4602)
  line L4446 (42.1411, 69.8819) -> (41.5628, 69.3036)
  line L4447 (48.26, 75.375) -> (48.26, 77.6325)
  line L4448 (48.26, 75.375) -> (48.26, 73.1175)
  line L4449 (48.26, 75.375) -> (49.4675, 75.375)
  line L4450 (48.26, 75.375) -> (47.0525, 75.375)
  line L4451 (63.31, 64.845) -> (63.31, 67.5425)
  line L4452 (63.31, 64.845) -> (63.31, 62.1475)
  line L4453 (63.31, 64.845) -> (64.7375, 64.845)
  line L4454 (63.31, 64.845) -> (61.8825, 64.845)
  line L4455 (69.778, 54.729) -> (57.078, 54.729)
  line L4456 (82.478, 54.729) -> (69.778, 54.729)
  line L4457 (96.81, 64.82) -> (94.543, 62.553)
  line L4458 (94.543, 62.553) -> (94.543, 54.729)
  line L4459 (94.543, 54.729) -> (57.078, 54.729)
  line L4460 (91.44, 76.2) -> (91.44, 69.215)
  line L4461 (95.835, 64.82) -> (96.81, 64.82)
  line L4462 (91.44, 69.215) -> (95.835, 64.82)
  line L4463 (3.52, 64.72) -> (4.79, 64.72)
  line L4464 (5.643, 63.867) -> (4.79, 64.72)
  line L4465 (5.643, 63.867) -> (5.643, 54.729)
  line L4466 (43.743, 54.729) -> (31.043, 54.729)
  line L4467 (31.043, 54.729) -> (31.5468, 54.729)
  line L4468 (31.5468, 54.729) -> (18.343, 54.729)
  line L4469 (18.343, 54.729) -> (18.9738, 54.729)
  line L4470 (18.9738, 54.729) -> (5.643, 54.729)
  line L4471 (3.52, 64.72) -> (8.89, 70.09)
  line L4472 (8.89, 70.09) -> (8.89, 76.835)
  line L4473 (18.8802, 54.729) -> (18.343, 54.729)
  line L4474 (18.8802, 54.729) -> (18.9738, 54.6354)
  line L4475 (18.9738, 54.6354) -> (18.9738, 54.729)
  line L4476 (31.5468, 54.3696) -> (31.5468, 54.6354)
  line L4477 (31.5468, 54.6354) -> (31.5468, 54.729)
  line L4478 (31.5468, 54.3696) -> (31.043, 54.729)
  line L4479 (48.26, 75.375) -> (48.26, 66.04)
  line L4480 (48.26, 66.04) -> (46.915, 64.695)
  line L4481 (46.915, 64.695) -> (37.02, 64.695)
  line L4482 (63.31, 64.845) -> (49.455, 64.845)
  line L4483 (49.455, 64.845) -> (48.26, 66.04)
  line L4484 (63.31, 64.845) -> (36.535, 64.845)
  line L4485 (37.17, 64.845) -> (37.02, 64.695)
  line L4486 (40.27, 64.845) -> (37.17, 64.845)
  line L4487 (37.17, 64.845) -> (36.535, 64.845)
  line L4488 (48.26, 75.375) -> (48.26, 72.835)
  line L4489 (56.25, 64.845) -> (63.31, 64.845)
  line L4490 (37.02, 64.695) -> (37.02, 64.7608)
  line L4491 (37.02, 64.7608) -> (42.1411, 69.8819)
  line L4492 (78.74, 76.2) -> (81.28, 76.2)
  line L4493 (21.59, 76.835) -> (19.05, 76.835)
  line L4494 (4.635, 15.875) -> (4.635, 30.721)
  line L4495 (4.635, 30.721) -> (5.643, 31.729)
  line L4496 (5.643, 31.729) -> (8.911, 31.729)
  line L4497 (8.911, 31.729) -> (10.16, 30.48)
  line L4498 (10.16, 20.32) -> (10.16, 16.51)
  line L4499 (20.955, 4.89) -> (20.955, 12.065)
  line L4500 (20.955, 12.065) -> (18.415, 14.605)
  line L4501 (18.415, 14.605) -> (18.415, 31.657)
  line L4502 (18.415, 31.657) -> (18.343, 31.729)
  line L4503 (18.343, 31.729) -> (21.611, 31.729)
  line L4504 (21.611, 31.729) -> (22.86, 30.48)
  line L4505 (22.86, 16.51) -> (22.86, 20.32)
  line L4506 (31.043, 12.772) -> (31.043, 31.729)
  line L4507 (33.655, 4.89) -> (33.655, 10.16)
  line L4508 (33.655, 10.16) -> (31.043, 12.772)
  line L4509 (31.043, 31.729) -> (34.311, 31.729)
  line L4510 (34.311, 31.729) -> (35.56, 30.48)
  line L4511 (35.56, 20.32) -> (35.56, 16.51)
  line L4512 (46.355, 4.89) -> (46.355, 9.525)
  line L4513 (46.355, 9.525) -> (43.18, 12.7)
  line L4514 (43.18, 31.1108) -> (43.815, 31.7458)
  line L4515 (43.18, 31.1108) -> (43.18, 12.7)
  line L4516 (43.743, 31.729) -> (47.011, 31.729)
  line L4517 (47.011, 31.729) -> (48.26, 30.48)
  line L4518 (43.815, 31.7458) -> (43.743, 31.729)
  line L4519 (48.26, 20.32) -> (46.355, 18.415)
  line L4520 (46.355, 18.415) -> (46.355, 16.51)
  line L4521 (53.34, 20.32) -> (57.15, 16.51)
  line L4522 (60.325, 28.482) -> (60.325, 5.525)
  line L4523 (60.325, 5.525) -> (59.69, 4.89)
  line L4524 (57.078, 31.729) -> (54.589, 31.729)
  line L4525 (54.589, 31.729) -> (53.34, 30.48)
  line L4526 (57.078, 31.729) -> (60.325, 28.482)
  line L4527 (67.31, 30.48) -> (68.487, 31.657)
  line L4528 (68.487, 31.657) -> (69.85, 31.657)
  line L4529 (72.39, 4.89) -> (72.39, 29.117)
  line L4530 (69.778, 31.729) -> (69.85, 31.657)
  line L4531 (72.39, 29.117) -> (69.85, 31.657)
  line L4532 (67.31, 20.32) -> (67.31, 16.51)
  line L4533 (84.455, 29.752) -> (84.455, 5.525)
  line L4534 (85.09, 4.89) -> (84.455, 5.525)
  line L4535 (78.74, 30.48) -> (79.917, 31.657)
  line L4536 (79.917, 31.657) -> (82.55, 31.657)
  line L4537 (82.55, 31.657) -> (84.455, 29.752)
  line L4538 (82.478, 31.729) -> (82.55, 31.657)
  line L4539 (78.74, 16.51) -> (78.74, 20.32)
  line L4540 (94.543, 31.729) -> (95.44, 30.832)
  line L4541 (95.44, 30.832) -> (95.44, 15.875)
  line L4542 (90.17, 30.48) -> (91.419, 31.729)
  line L4543 (91.419, 31.729) -> (94.543, 31.729)
  line L4544 (90.17, 20.32) -> (90.17, 16.51)
  line L4545 (34.9569, 77.0661) -> (34.7258, 76.835)
  line L4546 (34.7258, 76.835) -> (29.21, 76.835)
  line L4547 (35.75, 63.425) -> (35.75, 65.965)
  line L4548 (37.02, 62.155) -> (36.534, 62.2517)
  line L4549 (36.122, 66.863) -> (36.534, 67.1383)
  line L4550 (38.29, 65.965) -> (38.29, 63.425)
  line L4551 (36.534, 67.1383) -> (37.02, 67.235)
  line L4552 (37.918, 66.863) -> (38.1933, 66.451)
  line L4553 (35.8467, 62.939) -> (35.75, 63.425)
  line L4554 (37.918, 62.527) -> (37.506, 62.2517)
  line L4555 (37.02, 67.235) -> (37.506, 67.1383)
  line L4556 (37.506, 67.1383) -> (37.918, 66.863)
  line L4557 (38.1933, 62.939) -> (37.918, 62.527)
  line L4558 (38.1933, 66.451) -> (38.29, 65.965)
  line L4559 (35.8467, 66.451) -> (36.122, 66.863)
  line L4560 (36.122, 62.527) -> (35.8467, 62.939)
  line L4561 (37.506, 62.2517) -> (37.02, 62.155)
  line L4562 (36.534, 62.2517) -> (36.122, 62.527)
  line L4563 (35.75, 65.965) -> (35.8467, 66.451)
  line L4564 (38.29, 63.425) -> (38.1933, 62.939)
  line L4565 (2.622, 66.888) -> (3.034, 67.1633)
  line L4566 (4.6933, 62.964) -> (4.418, 62.552)
  line L4567 (2.3467, 66.476) -> (2.622, 66.888)
  line L4568 (3.034, 67.1633) -> (3.52, 67.26)
  line L4569 (3.52, 62.18) -> (3.034, 62.2767)
  line L4570 (4.6933, 66.476) -> (4.79, 65.99)
  line L4571 (4.006, 67.1633) -> (4.418, 66.888)
  line L4572 (2.3467, 62.964) -> (2.25, 63.45)
  line L4573 (3.034, 62.2767) -> (2.622, 62.552)
  line L4574 (4.418, 66.888) -> (4.6933, 66.476)
  line L4575 (2.25, 63.45) -> (2.25, 65.99)
  line L4576 (4.418, 62.552) -> (4.006, 62.2767)
  line L4577 (3.52, 67.26) -> (4.006, 67.1633)
  line L4578 (2.622, 62.552) -> (2.3467, 62.964)
  line L4579 (4.006, 62.2767) -> (3.52, 62.18)
  line L4580 (4.79, 63.45) -> (4.6933, 62.964)
  line L4581 (4.79, 65.99) -> (4.79, 63.45)
  line L4582 (2.25, 65.99) -> (2.3467, 66.476)
  line L4583 (64.58, 66.115) -> (64.58, 63.575)
  line L4584 (62.1367, 66.601) -> (62.412, 67.013)
  line L4585 (62.824, 67.2883) -> (63.31, 67.385)
  line L4586 (62.04, 66.115) -> (62.1367, 66.601)
  line L4587 (64.4833, 66.601) -> (64.58, 66.115)
  line L4588 (63.796, 67.2883) -> (64.208, 67.013)
  line L4589 (64.208, 67.013) -> (64.4833, 66.601)
  line L4590 (62.412, 67.013) -> (62.824, 67.2883)
  line L4591 (63.31, 67.385) -> (63.796, 67.2883)
  line L4592 (63.31, 62.305) -> (62.824, 62.4017)
  line L4593 (62.412, 62.677) -> (62.1367, 63.089)
  line L4594 (64.4833, 63.089) -> (64.208, 62.677)
  line L4595 (62.04, 63.575) -> (62.04, 66.115)
  line L4596 (62.1367, 63.089) -> (62.04, 63.575)
  line L4597 (64.58, 63.575) -> (64.4833, 63.089)
  line L4598 (63.796, 62.4017) -> (63.31, 62.305)
  line L4599 (64.208, 62.677) -> (63.796, 62.4017)
  line L4600 (62.824, 62.4017) -> (62.412, 62.677)
  line L4601 (97.708, 62.652) -> (97.296, 62.3767)
  line L4602 (96.324, 67.2633) -> (96.81, 67.36)
  line L4603 (96.324, 62.3767) -> (95.912, 62.652)
  line L4604 (98.08, 66.09) -> (98.08, 63.55)
  line L4605 (96.81, 67.36) -> (97.296, 67.2633)
  line L4606 (97.9833, 63.064) -> (97.708, 62.652)
  line L4607 (97.296, 67.2633) -> (97.708, 66.988)
  line L4608 (97.708, 66.988) -> (97.9833, 66.576)
  line L4609 (98.08, 63.55) -> (97.9833, 63.064)
  line L4610 (95.54, 66.09) -> (95.6367, 66.576)
  line L4611 (96.81, 62.28) -> (96.324, 62.3767)
  line L4612 (95.912, 62.652) -> (95.6367, 63.064)
  line L4613 (97.296, 62.3767) -> (96.81, 62.28)
  line L4614 (95.54, 63.55) -> (95.54, 66.09)
  line L4615 (95.912, 66.988) -> (96.324, 67.2633)
  line L4616 (95.6367, 66.576) -> (95.912, 66.988)
  line L4617 (95.6367, 63.064) -> (95.54, 63.55)
  line L4618 (97.9833, 66.576) -> (98.08, 66.09)
  line L4619 (7.811, 55.627) -> (8.0863, 55.215)
  line L4620 (4.373, 53.459) -> (3.887, 53.5557)
  line L4621 (3.1997, 55.215) -> (3.475, 55.627)
  line L4622 (6.913, 53.459) -> (4.373, 53.459)
  line L4623 (3.887, 55.9023) -> (4.373, 55.999)
  line L4624 (8.0863, 55.215) -> (8.183, 54.729)
  line L4625 (8.0863, 54.243) -> (7.811, 53.831)
  line L4626 (3.475, 55.627) -> (3.887, 55.9023)
  line L4627 (8.183, 54.729) -> (8.0863, 54.243)
  line L4628 (3.887, 53.5557) -> (3.475, 53.831)
  line L4629 (7.811, 53.831) -> (7.399, 53.5557)
  line L4630 (7.399, 55.9023) -> (7.811, 55.627)
  line L4631 (3.475, 53.831) -> (3.1997, 54.243)
  line L4632 (4.373, 55.999) -> (6.913, 55.999)
  line L4633 (7.399, 53.5557) -> (6.913, 53.459)
  line L4634 (6.913, 55.999) -> (7.399, 55.9023)
  line L4635 (3.103, 54.729) -> (3.1997, 55.215)
  line L4636 (3.1997, 54.243) -> (3.103, 54.729)
  line L4637 (3.887, 30.5557) -> (3.475, 30.831)
  line L4638 (4.373, 30.459) -> (3.887, 30.5557)
  line L4639 (3.887, 32.9023) -> (4.373, 32.999)
  line L4640 (4.373, 32.999) -> (6.913, 32.999)
  line L4641 (8.0863, 32.215) -> (8.183, 31.729)
  line L4642 (3.1997, 31.243) -> (3.103, 31.729)
  line L4643 (7.399, 32.9023) -> (7.811, 32.627)
  line L4644 (3.475, 30.831) -> (3.1997, 31.243)
  line L4645 (6.913, 32.999) -> (7.399, 32.9023)
  line L4646 (3.103, 31.729) -> (3.1997, 32.215)
  line L4647 (3.1997, 32.215) -> (3.475, 32.627)
  line L4648 (3.475, 32.627) -> (3.887, 32.9023)
  line L4649 (7.811, 32.627) -> (8.0863, 32.215)
  line L4650 (8.0863, 31.243) -> (7.811, 30.831)
  line L4651 (7.399, 30.5557) -> (6.913, 30.459)
  line L4652 (8.183, 31.729) -> (8.0863, 31.243)
  line L4653 (7.811, 30.831) -> (7.399, 30.5557)
  line L4654 (6.913, 30.459) -> (4.373, 30.459)
  line L4655 (20.883, 54.729) -> (20.7863, 54.243)
  line L4656 (19.613, 55.999) -> (20.099, 55.9023)
  line L4657 (16.175, 55.627) -> (16.587, 55.9023)
  line L4658 (15.8997, 55.215) -> (16.175, 55.627)
  line L4659 (15.803, 54.729) -> (15.8997, 55.215)
  line L4660 (20.7863, 55.215) -> (20.883, 54.729)
  line L4661 (20.511, 55.627) -> (20.7863, 55.215)
  line L4662 (20.511, 53.831) -> (20.099, 53.5557)
  line L4663 (20.099, 55.9023) -> (20.511, 55.627)
  line L4664 (17.073, 55.999) -> (19.613, 55.999)
  line L4665 (16.587, 55.9023) -> (17.073, 55.999)
  line L4666 (19.613, 53.459) -> (17.073, 53.459)
  line L4667 (20.099, 53.5557) -> (19.613, 53.459)
  line L4668 (16.175, 53.831) -> (15.8997, 54.243)
  line L4669 (20.7863, 54.243) -> (20.511, 53.831)
  line L4670 (15.8997, 54.243) -> (15.803, 54.729)
  line L4671 (17.073, 53.459) -> (16.587, 53.5557)
  line L4672 (16.587, 53.5557) -> (16.175, 53.831)
  line L4673 (15.803, 31.729) -> (15.8997, 32.215)
  line L4674 (16.587, 30.5557) -> (16.175, 30.831)
  line L4675 (17.073, 30.459) -> (16.587, 30.5557)
  line L4676 (20.7863, 31.243) -> (20.511, 30.831)
  line L4677 (20.511, 30.831) -> (20.099, 30.5557)
  line L4678 (16.175, 30.831) -> (15.8997, 31.243)
  line L4679 (20.511, 32.627) -> (20.7863, 32.215)
  line L4680 (20.883, 31.729) -> (20.7863, 31.243)
  line L4681 (17.073, 32.999) -> (19.613, 32.999)
  line L4682 (19.613, 32.999) -> (20.099, 32.9023)
  line L4683 (19.613, 30.459) -> (17.073, 30.459)
  line L4684 (20.7863, 32.215) -> (20.883, 31.729)
  line L4685 (20.099, 32.9023) -> (20.511, 32.627)
  line L4686 (16.175, 32.627) -> (16.587, 32.9023)
  line L4687 (16.587, 32.9023) -> (17.073, 32.999)
  line L4688 (15.8997, 32.215) -> (16.175, 32.627)
  line L4689 (15.8997, 31.243) -> (15.803, 31.729)
  line L4690 (20.099, 30.5557) -> (19.613, 30.459)
  line L4691 (29.287, 55.9023) -> (29.773, 55.999)
  line L4692 (32.799, 55.9023) -> (33.211, 55.627)
  line L4693 (33.4863, 54.243) -> (33.211, 53.831)
  line L4694 (28.875, 53.831) -> (28.5997, 54.243)
  line L4695 (32.313, 53.459) -> (29.773, 53.459)
  line L4696 (28.5997, 54.243) -> (28.503, 54.729)
  line L4697 (32.799, 53.5557) -> (32.313, 53.459)
  line L4698 (28.5997, 55.215) -> (28.875, 55.627)
  line L4699 (33.4863, 55.215) -> (33.583, 54.729)
  line L4700 (32.313, 55.999) -> (32.799, 55.9023)
  line L4701 (29.773, 53.459) -> (29.287, 53.5557)
  line L4702 (29.287, 53.5557) -> (28.875, 53.831)
  line L4703 (33.211, 55.627) -> (33.4863, 55.215)
  line L4704 (28.503, 54.729) -> (28.5997, 55.215)
  line L4705 (33.211, 53.831) -> (32.799, 53.5557)
  line L4706 (33.583, 54.729) -> (33.4863, 54.243)
  line L4707 (28.875, 55.627) -> (29.287, 55.9023)
  line L4708 (29.773, 55.999) -> (32.313, 55.999)
  line L4709 (28.5997, 31.243) -> (28.503, 31.729)
  line L4710 (33.4863, 32.215) -> (33.583, 31.729)
  line L4711 (33.211, 32.627) -> (33.4863, 32.215)
  line L4712 (29.773, 30.459) -> (29.287, 30.5557)
  line L4713 (28.875, 32.627) -> (29.287, 32.9023)
  line L4714 (33.583, 31.729) -> (33.4863, 31.243)
  line L4715 (28.875, 30.831) -> (28.5997, 31.243)
  line L4716 (32.313, 30.459) -> (29.773, 30.459)
  line L4717 (33.211, 30.831) -> (32.799, 30.5557)
  line L4718 (29.287, 32.9023) -> (29.773, 32.999)
  line L4719 (28.5997, 32.215) -> (28.875, 32.627)
  line L4720 (29.287, 30.5557) -> (28.875, 30.831)
  line L4721 (28.503, 31.729) -> (28.5997, 32.215)
  line L4722 (32.313, 32.999) -> (32.799, 32.9023)
  line L4723 (29.773, 32.999) -> (32.313, 32.999)
  line L4724 (32.799, 32.9023) -> (33.211, 32.627)
  line L4725 (33.4863, 31.243) -> (33.211, 30.831)
  line L4726 (32.799, 30.5557) -> (32.313, 30.459)
  line L4727 (45.499, 53.5557) -> (45.013, 53.459)
  line L4728 (41.575, 53.831) -> (41.2997, 54.243)
  line L4729 (41.987, 53.5557) -> (41.575, 53.831)
  line L4730 (45.911, 55.627) -> (46.1863, 55.215)
  line L4731 (41.203, 54.729) -> (41.2997, 55.215)
  line L4732 (42.473, 55.999) -> (45.013, 55.999)
  line L4733 (45.013, 53.459) -> (42.473, 53.459)
  line L4734 (42.473, 53.459) -> (41.987, 53.5557)
  line L4735 (45.499, 55.9023) -> (45.911, 55.627)
  line L4736 (41.2997, 55.215) -> (41.575, 55.627)
  line L4737 (41.987, 55.9023) -> (42.473, 55.999)
  line L4738 (46.1863, 54.243) -> (45.911, 53.831)
  line L4739 (45.013, 55.999) -> (45.499, 55.9023)
  line L4740 (41.575, 55.627) -> (41.987, 55.9023)
  line L4741 (41.2997, 54.243) -> (41.203, 54.729)
  line L4742 (46.283, 54.729) -> (46.1863, 54.243)
  line L4743 (46.1863, 55.215) -> (46.283, 54.729)
  line L4744 (45.911, 53.831) -> (45.499, 53.5557)
  line L4745 (45.499, 32.9023) -> (45.911, 32.627)
  line L4746 (41.203, 31.729) -> (41.2997, 32.215)
  line L4747 (41.575, 32.627) -> (41.987, 32.9023)
  line L4748 (42.473, 30.459) -> (41.987, 30.5557)
  line L4749 (41.987, 30.5557) -> (41.575, 30.831)
  line L4750 (41.2997, 31.243) -> (41.203, 31.729)
  line L4751 (46.1863, 31.243) -> (45.911, 30.831)
  line L4752 (45.911, 32.627) -> (46.1863, 32.215)
  line L4753 (46.1863, 32.215) -> (46.283, 31.729)
  line L4754 (41.575, 30.831) -> (41.2997, 31.243)
  line L4755 (41.2997, 32.215) -> (41.575, 32.627)
  line L4756 (45.013, 32.999) -> (45.499, 32.9023)
  line L4757 (41.987, 32.9023) -> (42.473, 32.999)
  line L4758 (45.013, 30.459) -> (42.473, 30.459)
  line L4759 (46.283, 31.729) -> (46.1863, 31.243)
  line L4760 (42.473, 32.999) -> (45.013, 32.999)
  line L4761 (45.911, 30.831) -> (45.499, 30.5557)
  line L4762 (45.499, 30.5557) -> (45.013, 30.459)
  line L4763 (58.348, 53.459) -> (55.808, 53.459)
  line L4764 (59.5213, 55.215) -> (59.618, 54.729)
  line L4765 (55.322, 55.9023) -> (55.808, 55.999)
  line L4766 (59.618, 54.729) -> (59.5213, 54.243)
  line L4767 (58.834, 53.5557) -> (58.348, 53.459)
  line L4768 (59.246, 55.627) -> (59.5213, 55.215)
  line L4769 (54.6347, 54.243) -> (54.538, 54.729)
  line L4770 (58.834, 55.9023) -> (59.246, 55.627)
  line L4771 (55.808, 55.999) -> (58.348, 55.999)
  line L4772 (59.246, 53.831) -> (58.834, 53.5557)
  line L4773 (54.91, 55.627) -> (55.322, 55.9023)
  line L4774 (58.348, 55.999) -> (58.834, 55.9023)
  line L4775 (55.322, 53.5557) -> (54.91, 53.831)
  line L4776 (54.91, 53.831) -> (54.6347, 54.243)
  line L4777 (59.5213, 54.243) -> (59.246, 53.831)
  line L4778 (54.6347, 55.215) -> (54.91, 55.627)
  line L4779 (54.538, 54.729) -> (54.6347, 55.215)
  line L4780 (55.808, 53.459) -> (55.322, 53.5557)
  line L4781 (58.834, 30.5557) -> (58.348, 30.459)
  line L4782 (54.6347, 32.215) -> (54.91, 32.627)
  line L4783 (54.91, 32.627) -> (55.322, 32.9023)
  line L4784 (54.91, 30.831) -> (54.6347, 31.243)
  line L4785 (54.538, 31.729) -> (54.6347, 32.215)
  line L4786 (59.5213, 32.215) -> (59.618, 31.729)
  line L4787 (55.322, 30.5557) -> (54.91, 30.831)
  line L4788 (54.6347, 31.243) -> (54.538, 31.729)
  line L4789 (59.246, 30.831) -> (58.834, 30.5557)